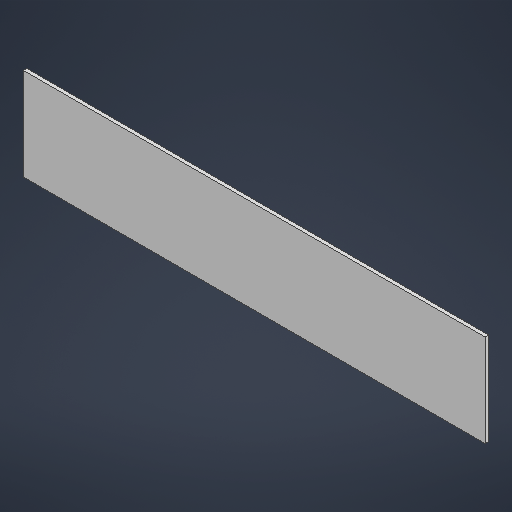
# Autodesk Inventor part: Tapa lados
Saved by Autodesk Inventor 2026 (Build 300175050, 175E)
## iProperties
Created: 2025-10-07
Part Number: Tapa lados
Material: Generic
Document SubType Name: Modeling
Designer: habbo
Density: 1 g/cm^3
Appearance: Default
Author: habbo
Autodesk Inventor part; units mm, degrees
ref_plane "YZ Plane" through (0, 0, 0) normal (1, 0, 0) x (0, 1, 0)
ref_plane "XZ Plane" through (0, 0, 0) normal (0, 1, 0) x (-1, 0, 0)
ref_plane "XY Plane" through (0, 0, 0) normal (0, 0, 1) x (1, 0, 0)
sketch "Sketch1" plane through (0, 0, 0) normal (0, 0, 1) x (1, 0, 0)
  line L0 (-200, -40) -> (200, -40)
  line L1 (200, -40) -> (200, 40)
  line L2 (200, 40) -> (-200, 40)
  line L3 (-200, 40) -> (-200, -40)
  line L4 (-200, -40) -> (200, 40) construction
  line L5 (200, -40) -> (-200, 40) construction
  point P0 (0, 0)
  dimension "d0" = 400
  dimension "d1" = 80
  constraints: 12 end point, 2 midpoint, 2 parallel, 1 horizontal, 1 perpendicular
  measures "d0" distance of L2.end L1.end
  measures "d1" distance of L1.end L0.end
extrude "Extrusion1" add sketch "Sketch1" along normal mid plane 3
body "Solid1"
